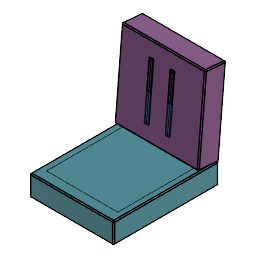
Smart_Chair (Autodesk Fusion 360 design; units mm, degrees)
part number: 2026-02-20-20-56-46-946
part number: 2026-02-20-20-58-49-113
part number: 2026-02-24-11-41-41-423
part number: 2026-02-24-11-48-27-673
part number: 2026-02-24-12-03-58-197
part number: 2026-02-24-12-17-04-515
Autodesk Fusion 360 part; units mm, degrees
sketch "Sketch1" plane through (0, 0, 0) normal (0, 0, 1) x (1, 0, 0) in component "Smart_Sprayer_Corner_Safety_Mount"
  line L0 (-12.6, 12.6) -> (12.6, 12.6) construction
  line L1 (12.6, 12.6) -> (12.6, -12.6) construction
  line L2 (12.6, -12.6) -> (-12.6, -12.6) construction
  line L3 (-12.6, -12.6) -> (-12.6, 12.6) construction
  line L4 (-12.6, 12.6) -> (12.6, -12.6) construction
  line L5 (12.6, 12.6) -> (-12.6, -12.6) construction
  line L6 (-12.6, 12.6) -> (-14.6, 12.6)
  line L7 (-14.6, 12.6) -> (-14.6, -12.6)
  line L8 (-14.6, -12.6) -> (-12.6, -12.6)
  line L9 (-12.6, -12.6) -> (-12.6, 12.6)
  line L10 (-14.6, -12.6) -> (12.6, -12.6)
  line L11 (12.6, -12.6) -> (12.6, -14.6)
  line L12 (12.6, -14.6) -> (-14.6, -14.6)
  line L13 (-14.6, -14.6) -> (-14.6, -12.6)
  dimension "d1" = 25.2
  dimension "d2" = 25.2
  dimension "d3" = 2
  dimension "d4" = 2
  constraint horizontal L0
  constraint perpendicular L0 L1
  constraint parallel L0 L2
  constraint parallel L1 L3
  constraint coincident L4 origin
  constraint coincident L5 origin
  constraint horizontal L6
  constraint vertical L7
  constraint horizontal L8
  constraint vertical L9
  constraint horizontal L10
  constraint vertical L11
  constraint horizontal L12
  constraint vertical L13
  measures "d1" distance of L1.end L2.end
  measures "d2" distance of L0.end L1.end
  measures "d3" distance of L0.start L6.end
  measures "d4" distance of L7.end L12.end
extrude "Extrude1" add sketch "Sketch1" along normal blind 27.2 makes body 1 in component "Smart_Sprayer_Corner_Safety_Mount"
sketch "Sketch2" plane through (0, -12.6, 0) normal (0, 1, 0) x (-1, 0, 0) in component "Smart_Sprayer_Corner_Safety_Mount"
  line L0 (-12.6, 0) -> (12.6, 0)
  line L1 (12.6, 0) -> (12.6, 27.2)
  line L2 (12.6, 27.2) -> (-12.6, 27.2)
  line L3 (-12.6, 27.2) -> (-12.6, 0)
  line L4 (-12.6, 27.2) -> (12.6, 27.2)
  line L5 (12.6, 27.2) -> (12.6, 25.2)
  line L6 (12.6, 25.2) -> (-12.6, 25.2)
  line L7 (-12.6, 25.2) -> (-12.6, 27.2)
  dimension "d7" = 2
  constraint horizontal L4
  constraint vertical L5
  constraint horizontal L6
  constraint vertical L7
  constraint coincident L2.end L3.start
  measures "d7" distance of L2.end L6.end
extrude "Extrude2" add sketch "Sketch2" along normal blind 25.2 contours L1 L2 L3 L4 L5 L6 L7 bodies 1 in component "Smart_Sprayer_Corner_Safety_Mount"
fillet "Fillet1" radius 1.25 9 edges at (-14.6, -1, 27.2) (-1, -14.6, 27.2) (-14.6, -14.6, 13.6) (12.6, -14.6, 13.6) (-1, 12.6, 27.2) (-14.6, -1, 0) (-14.6, 12.6, 13.6) (12.6, -1, 27.2) (-1, -14.6, 0) on bodies 1 in component "Smart_Sprayer_Corner_Safety_Mount"
sketch "Sketch1 (2)" plane through (0, 0, 0) normal (0, 1, 0) x (1, 0, 0) in component "Smart_Chair_Cushion_Back"
  line L0 (200, 200) -> (-200, 200)
  line L1 (-200, 200) -> (-200, -200)
  line L2 (-200, -200) -> (200, -200)
  line L3 (200, -200) -> (200, 200)
  line L4 (200, 200) -> (-200, -200) construction
  line L5 (-200, 200) -> (200, -200) construction
  dimension "d12" = 400
  dimension "d13" = 400
  constraint horizontal L0
  constraint perpendicular L0 L1
  constraint parallel L0 L2
  constraint parallel L1 L3
  constraint coincident L4 origin
  constraint coincident L5 origin
  measures "d12" distance of L1.end L2.end
  measures "d13" distance of L0.end L1.end
extrude "Extrude1'" add sketch "Sketch1 (2)" against normal blind 100 separate body makes body 2 in component "Smart_Chair_Cushion_Back"
fillet "Fillet1'" radius 5 6 faces at (-66.6667, -100, -66.6667) (-66.6667, -33.3333, 200) (200, -33.3333, 66.6667) (-66.6667, 0, -66.6667) (-200, -33.3333, -66.6667) (66.6667, -33.3333, -200) on bodies 2 in component "Smart_Chair_Cushion_Back"
sketch "Sketch1 (3)" plane through (0, -100, 0) normal (0, -1, 0) x (1, 0, 0) in component "Smart_Chair_Cushion_Back_Sensor_Mount"
  line L0 (195, 195) -> (-195, 195)
  line L1 (-195, 195) -> (-195, -195)
  line L2 (-195, -195) -> (195, -195)
  line L3 (195, -195) -> (195, 195)
  line L4 (-50, 195) -> (50, 195) construction
  line L5 (50, 195) -> (50, -195) construction
  line L6 (50, -195) -> (-50, -195) construction
  line L7 (-50, -195) -> (-50, 195) construction
  line L8 (-50, 195) -> (50, -195) construction
  line L9 (50, 195) -> (-50, -195) construction
  line L10 (0, 0) -> (0, 130) construction
  line L11 (0, 130) -> (-50, 130) construction
  line L12 (-50, 0) -> (-40, 0)
  line L13 (-40, 0) -> (-40, 130)
  line L14 (-40, 130) -> (-50, 130)
  line L15 (-50, 130) -> (-50, 0)
  line L16 (-50, 0) -> (-60, 0)
  line L17 (-60, 0) -> (-60, 130)
  line L18 (-60, 130) -> (-50, 130)
  line L19 (-50, 130) -> (-50, 0)
  dimension "d18" = 100
  dimension "d19" = 130
  dimension "d20" = 10
  dimension "d21" = 130
  dimension "d22" = 10
  dimension "d23" = 130
  constraint horizontal L4
  constraint perpendicular L4 L5
  constraint parallel L4 L6
  constraint parallel L5 L7
  constraint coincident L8 L10.start
  constraint coincident L9 L10.start
  constraint coincident L10.start origin
  constraint parallel L5 L10
  constraint coincident L7 L11.end
  constraint perpendicular L7 L11
  constraint horizontal L12
  constraint vertical L13
  constraint horizontal L14
  constraint vertical L15
  constraint midpoint L7 L12.start
  constraint horizontal L16
  constraint vertical L17
  constraint horizontal L18
  constraint vertical L19
  measures "d18" distance of L5.end L6.end
  measures "d19" distance of L10.start L10.end
  measures "d20" distance of L12.start L12.end
  measures "d21" distance of L12.start L11.end
  measures "d22" distance of L12.start L16.end
  measures "d23" distance of L12.start L11.end
extrude "Extrude1''" add sketch "Sketch1 (3)" along normal blind 3 separate body contours L12 L13 L14 L15 L19 | L15 L16 L17 L18 L19 makes body 3 in component "Smart_Chair_Cushion_Back_Sensor_Mount"
shell "Shell1" thickness 0.6 removed faces 2 at (-43.3333, -101, 130) at (-56.6667, -101, 130) on bodies 3 in component "Smart_Chair_Cushion_Back_Sensor_Mount"
sketch "Sketch2 (2)" plane through (0, -100, 0) normal (0, 1, 0) x (-1, 0, 0) in component "Smart_Chair_Cushion_Back_Sensor_Mount"
  line L0 (40, 0) -> (60, 0)
  line L1 (60, 0) -> (60, 130)
  line L2 (60, 130) -> (40, 130)
  line L3 (40, 130) -> (40, 0)
  line L4 (40, 130) -> (41, 130)
  line L5 (60, 130) -> (59, 130)
  line L6 (41, 130) -> (49, 130)
  line L7 (49, 130) -> (49, 0)
  line L8 (49, 0) -> (41, 0)
  line L9 (41, 0) -> (41, 130)
  line L10 (59, 130) -> (51, 130)
  line L11 (51, 130) -> (51, 0)
  line L12 (51, 0) -> (59, 0)
  line L13 (59, 0) -> (59, 130)
  dimension "d27" = 1
  dimension "d28" = 1
  dimension "d29" = 8
  dimension "d30" = 8
  constraint coincident L2.end L3.start
  constraint perpendicular L3 L4
  constraint coincident L1.end L2.start
  constraint perpendicular L1 L5
  constraint horizontal L6
  constraint vertical L7
  constraint horizontal L8
  constraint vertical L9
  constraint horizontal L10
  constraint vertical L11
  constraint horizontal L12
  constraint vertical L13
  measures "d27" distance of L2.end L4.end
  measures "d28" distance of L1.end L5.end
  measures "d29" distance of L4.end L6.end
  measures "d30" distance of L5.end L10.end
extrude "Extrude2'" add sketch "Sketch2 (2)" along normal blind 0.3 separate body contours L0 L2 L6 L7 L8 L9 | L0 L2 L10 L11 L12 L13 makes body 4 at (-43.6667, -100, 43.3333) makes body 5 at (-53.6667, -100, 43.3333) in component "Smart_Chair_Cushion_Back_Sensor_Mount"
chamfer "Chamfer1" distance 0.9 distance2 0.9 8 edges at (-40, -103, 65) (-40, -100, 65) (-40.6, -100.6, 65.3) (-40.6, -102.4, 65.3) (-59.4, -100.6, 65.3) (-59.4, -102.4, 65.3) (-60, -100, 65) (-60, -103, 65) measured on face at (-53.3333, -103, 86.6667) measured on face at (-40, -101, 43.3333) measured on face at (-53.1333, -100.6, 43.7333) measured on face at (-40.6, -101.8, 43.7333) measured on face at (-59.4, -101.8, 43.7333) measured on face at (-59.4, -101.8, 43.7333) measured on face at (-53.3333, -100, 86.6667) measured on face at (-53.3333, -103, 86.6667) on bodies 3 in component "Smart_Chair_Cushion_Back_Sensor_Mount"
sketch "Sketch3" plane through (0, -100, 0) normal (0, 1, 0) x (-1, 0, 0) in component "Smart_Chair_Cushion_Back_Sensor_Mount"
  line L0 (59.1, 0) -> (59.1, 130)
  line L1 (59.1, 130) -> (40.9, 130)
  line L2 (40.9, 130) -> (40.9, 0)
  line L3 (40.9, 0) -> (59.1, 0)
  line L4 (55, 125) -> (45, 125)
  line L5 (45, 125) -> (45, 135)
  line L6 (45, 135) -> (55, 135)
  line L7 (55, 135) -> (55, 125)
  line L8 (55, 125) -> (45, 135) construction
  line L9 (45, 125) -> (55, 135) construction
  point P0 (50, 130)
  dimension "d35" = 10
  dimension "d36" = 10
  constraint horizontal L4
  constraint perpendicular L4 L5
  constraint parallel L4 L6
  constraint parallel L5 L7
  constraint coincident L8 P0
  constraint coincident L9 P0
  constraint midpoint L1 P0
  measures "d35" distance of L5.end L6.end
  measures "d36" distance of L4.end L5.end
extrude "Extrude3" cut sketch "Sketch3" along normal mid plane 4 contours L1 L4 L5 L7 bodies 3 in component "Smart_Chair_Cushion_Back_Sensor_Mount"
pattern_linear "00000000-0000-0000-0000-000000000000" [suppressed]
sketch "Sketch1 (4)" plane through (0, -100, 0) normal (0, -1, 0) x (1, 0, 0) in component "Smart_Chair_Cushion_Back_Sensor_Mount (1)"
  line L0 (195, 195) -> (-195, 195)
  line L1 (-195, 195) -> (-195, -195)
  line L2 (-195, -195) -> (195, -195)
  line L3 (195, -195) -> (195, 195)
  line L4 (-50, 195) -> (50, 195) construction
  line L5 (50, 195) -> (50, -195) construction
  line L6 (50, -195) -> (-50, -195) construction
  line L7 (-50, -195) -> (-50, 195) construction
  line L8 (-50, 195) -> (50, -195) construction
  line L9 (50, 195) -> (-50, -195) construction
  line L10 (0, 0) -> (0, 130) construction
  line L11 (0, 130) -> (-50, 130) construction
  line L12 (-50, 0) -> (-40, 0)
  line L13 (-40, 0) -> (-40, 130)
  line L14 (-40, 130) -> (-50, 130)
  line L15 (-50, 130) -> (-50, 0)
  line L16 (-50, 0) -> (-60, 0)
  line L17 (-60, 0) -> (-60, 130)
  line L18 (-60, 130) -> (-50, 130)
  line L19 (-50, 130) -> (-50, 0)
  dimension "d18_1" = 100
  dimension "d19_1" = 130
  dimension "d20_1" = 10
  dimension "d21_1" = 130
  dimension "d22_1" = 10
  dimension "d23_1" = 130
  constraint horizontal L4
  constraint perpendicular L4 L5
  constraint parallel L4 L6
  constraint parallel L5 L7
  constraint coincident L8 L10.start
  constraint coincident L9 L10.start
  constraint coincident L10.start origin
  constraint parallel L5 L10
  constraint coincident L7 L11.end
  constraint perpendicular L7 L11
  constraint horizontal L12
  constraint vertical L13
  constraint horizontal L14
  constraint vertical L15
  constraint midpoint L7 L12.start
  constraint horizontal L16
  constraint vertical L17
  constraint horizontal L18
  constraint vertical L19
  measures "d18_1" distance of L5.end L6.end
  measures "d19_1" distance of L10.start L10.end
  measures "d20_1" distance of L12.start L12.end
  measures "d21_1" distance of L12.start L11.end
  measures "d22_1" distance of L12.start L16.end
  measures "d23_1" distance of L12.start L11.end
extrude "Extrude1'''" add sketch "Sketch1 (4)" along normal blind 3 separate body contours L12 L13 L14 L15 L19 | L15 L16 L17 L18 L19 makes body 6 in component "Smart_Chair_Cushion_Back_Sensor_Mount (1)"
shell "Shell1'" thickness 0.6 removed faces 2 at (-43.3333, -101, 130) at (-56.6667, -101, 130) on bodies 6 in component "Smart_Chair_Cushion_Back_Sensor_Mount (1)"
sketch "Sketch2 (3)" plane through (0, -100, 0) normal (0, 1, 0) x (-1, 0, 0) in component "Smart_Chair_Cushion_Back_Sensor_Mount (1)"
  line L0 (40, 0) -> (60, 0)
  line L1 (60, 0) -> (60, 130)
  line L2 (60, 130) -> (40, 130)
  line L3 (40, 130) -> (40, 0)
  line L4 (40, 130) -> (41, 130)
  line L5 (60, 130) -> (59, 130)
  line L6 (41, 130) -> (49, 130)
  line L7 (49, 130) -> (49, 0)
  line L8 (49, 0) -> (41, 0)
  line L9 (41, 0) -> (41, 130)
  line L10 (59, 130) -> (51, 130)
  line L11 (51, 130) -> (51, 0)
  line L12 (51, 0) -> (59, 0)
  line L13 (59, 0) -> (59, 130)
  dimension "d27_1" = 1
  dimension "d28_1" = 1
  dimension "d29_1" = 8
  dimension "d30_1" = 8
  constraint coincident L2.end L3.start
  constraint perpendicular L3 L4
  constraint coincident L1.end L2.start
  constraint perpendicular L1 L5
  constraint horizontal L6
  constraint vertical L7
  constraint horizontal L8
  constraint vertical L9
  constraint horizontal L10
  constraint vertical L11
  constraint horizontal L12
  constraint vertical L13
  measures "d27_1" distance of L2.end L4.end
  measures "d28_1" distance of L1.end L5.end
  measures "d29_1" distance of L4.end L6.end
  measures "d30_1" distance of L5.end L10.end
extrude "Extrude2''" add sketch "Sketch2 (3)" along normal blind 0.3 separate body contours L0 L2 L6 L7 L8 L9 | L0 L2 L10 L11 L12 L13 makes body 7 at (-43.6667, -100, 43.3333) makes body 8 at (-53.6667, -100, 43.3333) in component "Smart_Chair_Cushion_Back_Sensor_Mount (1)"
chamfer "Chamfer1'" distance 0.9 distance2 0.9 8 edges at (-40, -103, 65) (-40, -100, 65) (-40.6, -100.6, 65.3) (-40.6, -102.4, 65.3) (-59.4, -100.6, 65.3) (-59.4, -102.4, 65.3) (-60, -100, 65) (-60, -103, 65) measured on face at (-53.3333, -103, 86.6667) measured on face at (-40, -101, 43.3333) measured on face at (-53.1333, -100.6, 43.7333) measured on face at (-40.6, -101.8, 43.7333) measured on face at (-59.4, -101.8, 43.7333) measured on face at (-59.4, -101.8, 43.7333) measured on face at (-53.3333, -100, 86.6667) measured on face at (-53.3333, -103, 86.6667) on bodies 6 in component "Smart_Chair_Cushion_Back_Sensor_Mount (1)"
sketch "Sketch3 (2)" plane through (0, -100, 0) normal (0, 1, 0) x (-1, 0, 0) in component "Smart_Chair_Cushion_Back_Sensor_Mount (1)"
  line L0 (59.1, 0) -> (59.1, 130)
  line L1 (59.1, 130) -> (40.9, 130)
  line L2 (40.9, 130) -> (40.9, 0)
  line L3 (40.9, 0) -> (59.1, 0)
  line L4 (55, 125) -> (45, 125)
  line L5 (45, 125) -> (45, 135)
  line L6 (45, 135) -> (55, 135)
  line L7 (55, 135) -> (55, 125)
  line L8 (55, 125) -> (45, 135) construction
  line L9 (45, 125) -> (55, 135) construction
  point P0 (50, 130)
  dimension "d35_1" = 10
  dimension "d36_1" = 10
  constraint horizontal L4
  constraint perpendicular L4 L5
  constraint parallel L4 L6
  constraint parallel L5 L7
  constraint coincident L8 P0
  constraint coincident L9 P0
  constraint midpoint L1 P0
  measures "d35_1" distance of L5.end L6.end
  measures "d36_1" distance of L4.end L5.end
extrude "Extrude3'" cut sketch "Sketch3 (2)" along normal mid plane 4 contours L1 L4 L5 L7 bodies 6 in component "Smart_Chair_Cushion_Back_Sensor_Mount (1)"
sketch "Sketch4" plane through (0, -103, 0) normal (0, -1, 0) x (1, 0, 0) in component "Smart_Chair_Cushion_Back_Sensor_Mount (1)"
  line L0 (-59.1, 130) -> (-59.1, 0)
  line L1 (-59.1, 0) -> (-40.9, 0)
  line L2 (-40.9, 0) -> (-40.9, 130)
  line L3 (-40.9, 130) -> (-59.1, 130)
pattern_linear "00000000-0000-0000-0000-000000000000'" [suppressed]
sketch "Sketch2 (4)" plane through (0, -100, 0) normal (0, -1, 0) x (1, 0, 0) in component "Smart_Chair_Cushion_Back"
  line L0 (195, 195) -> (-195, 195)
  line L1 (-195, 195) -> (-195, -195)
  line L2 (-195, -195) -> (195, -195)
  line L3 (195, -195) -> (195, 195)
  line L4 (-50, 195) -> (50, 195) construction
  line L5 (50, 195) -> (50, -195) construction
  line L6 (50, -195) -> (-50, -195) construction
  line L7 (-50, -195) -> (-50, 195) construction
  line L8 (-50, 195) -> (50, -195) construction
  line L9 (50, 195) -> (-50, -195) construction
  line L10 (-47.1154, 122.5) -> (47.1154, 122.5) construction
  line L11 (47.1154, 122.5) -> (47.1154, -122.5) construction
  line L12 (47.1154, -122.5) -> (-47.1154, -122.5) construction
  line L13 (-47.1154, -122.5) -> (-47.1154, 122.5) construction
  line L14 (-47.1154, 122.5) -> (47.1154, -122.5) construction
  line L15 (47.1154, 122.5) -> (-47.1154, -122.5) construction
  circle A0 centre (-50, 122.5) radius 2
  circle A1 centre (50, 122.5) radius 2
  circle A2 centre (-50, -122.5) radius 2
  circle A3 centre (50, -122.5) radius 2
  dimension "d47" = 100
  dimension "d48" = 245
  dimension "d49" = 4
  dimension "d50" = 4
  dimension "d51" = 4
  dimension "d52" = 4
  constraint horizontal L4
  constraint perpendicular L4 L5
  constraint parallel L4 L6
  constraint parallel L5 L7
  constraint coincident L8 origin
  constraint coincident L9 origin
  constraint horizontal L10
  constraint perpendicular L10 L11
  constraint parallel L10 L12
  constraint parallel L11 L13
  constraint coincident L14 origin
  constraint coincident L15 origin
  constraint coincident L7 A0.centre
  constraint coincident L5 A1.centre
  constraint coincident L7 A2.centre
  constraint coincident L5 A3.centre
  measures "d47" distance of L5.end L6.end
  measures "d48" distance of L10.end L11.end
  measures "d49" diameter of A0
  measures "d50" diameter of A1
  measures "d51" diameter of A2
  measures "d52" diameter of A3
extrude "Extrude2'''" cut sketch "Sketch2 (4)" against normal blind 10 contours A0 | A1 | A2 | A3 bodies 2 in component "Smart_Chair_Cushion_Back"
sketch "Sketch3 (3)" plane through (0, 0, 0) normal (1, 0, 0) x (0, 1, 0) in component "Smart_Chair_Cushion_Back"
sketch "Sketch4 (2)" plane through (-200, 0, 0) normal (-1, 0, 0) x (0, -1, 0) in component "Smart_Chair_Cushion_Back"
  line L0 (5, -195) -> (95, -195)
  line L1 (95, -195) -> (95, 195)
  line L2 (95, 195) -> (5, 195)
  line L3 (5, 195) -> (5, -195)
  line L4 (50, 195) -> (50, 95) construction
  line L5 (50, -195) -> (50, -95) construction
  circle A0 centre (50, -95) radius 2 construction
  circle A1 centre (50, 95) radius 2
  circle A2 centre (50, -95) radius 2
  dimension "d55" = 100
  dimension "d56" = 100
  dimension "d57" = 4
  dimension "d58" = 4
  dimension "d59" = 4
  constraint vertical L4
  constraint midpoint L2 L4.start
  constraint midpoint L0 L5.start
  constraint perpendicular L0 L5
  constraint coincident L5.end A0.centre
  constraint coincident L4.end A1.centre
  measures "d55" distance of L4.start L4.end
  measures "d56" distance of L5.start L5.end
  measures "d57" diameter of A0
  measures "d58" diameter of A1
  measures "d59" diameter of A2
extrude "Extrude3''" cut sketch "Sketch4 (2)" against normal blind 10 contours A1 | A2 bodies 2 in component "Smart_Chair_Cushion_Back"
sketch "Sketch5" plane through (-200, 0, 0) normal (-1, 0, 0) x (0, -1, 0) in component "Smart_Chair_Cushion_Back"
  circle A0 centre (50, 95) radius 2
  circle A1 centre (50, -95) radius 2
  line L0 (5, -195) -> (95, -195)
  line L1 (95, -195) -> (95, 195)
  line L2 (95, 195) -> (5, 195)
  line L3 (5, 195) -> (5, -195)
  line L4 (50, 95) -> (50, -95) construction
  line L5 (0, 50) -> (100, 50) construction
  line L6 (100, 50) -> (100, -50) construction
  line L7 (100, -50) -> (0, -50) construction
  line L8 (0, -50) -> (0, 50) construction
  line L9 (0, 50) -> (100, -50) construction
  line L10 (100, 50) -> (0, -50) construction
  line L11 (20, 50) -> (80, 50) construction
  line L12 (80, 50) -> (80, -50) construction
  line L13 (80, -50) -> (20, -50) construction
  line L14 (20, -50) -> (20, 50) construction
  line L15 (20, 50) -> (80, -50) construction
  line L16 (80, 50) -> (20, -50) construction
  line L17 (20, 50) -> (30, 50)
  line L18 (30, 50) -> (30, -50)
  line L19 (30, -50) -> (20, -50)
  line L20 (20, -50) -> (20, 50)
  line L21 (20, 50) -> (10, 50)
  line L22 (10, 50) -> (10, -50)
  line L23 (10, -50) -> (20, -50)
  line L24 (20, -50) -> (20, 50)
  line L25 (80, 50) -> (70, 50)
  line L26 (70, 50) -> (70, -50)
  line L27 (70, -50) -> (80, -50)
  line L28 (80, -50) -> (80, 50)
  line L29 (80, 50) -> (90, 50)
  line L30 (90, 50) -> (90, -50)
  line L31 (90, -50) -> (80, -50)
  line L32 (80, -50) -> (80, 50)
  point P0 (50, 0)
  point P1 (50, 0)
  dimension "d62" = 100
  dimension "d63" = 100
  dimension "d64" = 60
  dimension "d65" = 10
  constraint coincident A0.centre L4.start
  constraint coincident A1.centre L4.end
  constraint horizontal L5
  constraint perpendicular L5 L6
  constraint parallel L5 L7
  constraint parallel L6 L8
  constraint coincident L9 P1
  constraint coincident L10 P1
  constraint midpoint L4 P1
  constraint horizontal L11
  constraint perpendicular L11 L12
  constraint parallel L11 L13
  constraint parallel L12 L14
  constraint coincident L15 P1
  constraint coincident L16 P1
  constraint coincident P1 P0
  constraint horizontal L17
  constraint vertical L18
  constraint horizontal L19
  constraint vertical L20
  constraint horizontal L21
  constraint vertical L22
  constraint horizontal L23
  constraint vertical L24
  constraint coincident L7 L22.end
  constraint horizontal L25
  constraint vertical L26
  constraint horizontal L27
  constraint vertical L28
  constraint coincident L7 L26.end
  constraint horizontal L29
  constraint vertical L30
  constraint horizontal L31
  constraint vertical L32
  constraint coincident L7 L30.end
  measures "d62" distance of L6.end L7.end
  measures "d63" distance of L5.end L6.end
  measures "d64" distance of L12.end L13.end
  measures "d65" distance of L11.start L17.end
extrude "Extrude4" add sketch "Sketch5" along normal blind 0.3 separate body contours L17 L18 L19 L20 L24 | L20 L21 L22 L23 L24 | L25 L26 L27 L28 L32 | L28 L29 L30 L31 L32 makes body 9 at (-200, -16.6667, 16.6667) makes body 10 at (-200, -83.3333, -16.6667) in component "Smart_Chair_Cushion_Back"
sketch "Sketch1 (5)" plane through (0, 0, 0) normal (0, 0, 1) x (1, 0, 0) in component "Smart_Chair_Cushion_Sit"
  line L0 (0, -120) -> (0, -520) construction
  line L1 (-200, -520) -> (200, -520)
  line L2 (200, -520) -> (200, -120)
  line L3 (200, -120) -> (-200, -120)
  line L4 (-200, -120) -> (-200, -520)
  line L5 (-200, -520) -> (200, -120) construction
  line L6 (200, -520) -> (-200, -120) construction
  point P0 (0, -320)
  dimension "d68" = 400
  dimension "d69" = 400
  dimension "d70" = 400
  constraint vertical L0
  constraint horizontal L1
  constraint perpendicular L1 L2
  constraint parallel L1 L3
  constraint parallel L2 L4
  constraint coincident L5 P0
  constraint coincident L6 P0
  constraint midpoint L0 P0
  measures "d68" distance of L0.start L0.end
  measures "d69" distance of L2.end L3.end
  measures "d70" distance of L1.end L2.end
extrude "Extrude1''''" add sketch "Sketch1 (5)" against normal blind 300 separate body makes body 11 in component "Smart_Chair_Cushion_Sit"
extrude "Extrude2''''" cut 1 faces at (-66.6667, -253.3333, 0) along direction (0, 0, -1) blind 200 on bodies 11 bodies 11 in component "Smart_Chair_Cushion_Sit"
extrude "Extrude3'''" add 1 faces at (66.6667, -120, -233.3333) along direction (0, 1, 0) blind 100 on bodies 11 bodies 11 in component "Smart_Chair_Cushion_Sit"
fillet "Fillet1''" radius 5 1 edges at (-200, -270, -300) 6 faces at (200, -186.6667, -266.6667) (66.6667, -20, -233.3333) (-66.6667, -520, -233.3333) (-66.6667, -186.6667, -200) (-200, -353.3333, -233.3333) (-66.6667, -186.6667, -300) on bodies 11 in component "Smart_Chair_Cushion_Sit"
sketch "Sketch2 (5)" plane through (0, 0, -300) normal (0, 0, -1) x (1, 0, 0) in component "Smart_Chair_Cushion_Sit"
  line L0 (-195, 515) -> (-195, 25)
  line L1 (-195, 25) -> (195, 25)
  line L2 (195, 25) -> (195, 515)
  line L3 (195, 515) -> (-195, 515)
  line L4 (-195, 515) -> (195, 25) construction
  line L5 (-170, 470) -> (170, 470)
  line L6 (170, 470) -> (170, 70)
  line L7 (170, 70) -> (-170, 70)
  line L8 (-170, 70) -> (-170, 470)
  line L9 (-170, 470) -> (170, 70) construction
  line L10 (170, 470) -> (-170, 70) construction
  point P0 (0, 270)
  dimension "d79" = 340
  dimension "d80" = 400
  constraint coincident L0.start L3.end
  constraint coincident L1.end L2.start
  constraint horizontal L5
  constraint perpendicular L5 L6
  constraint parallel L5 L7
  constraint parallel L6 L8
  constraint coincident L9 P0
  constraint coincident L10 P0
  constraint midpoint L4 P0
  measures "d79" distance of L6.end L7.end
  measures "d80" distance of L5.end L6.end
extrude "Extrude4'" cut sketch "Sketch2 (5)" against normal blind 97 contours L5 L6 L7 L8 bodies 11 in component "Smart_Chair_Cushion_Sit"
component "Smart_Sprayer_Corner_Safety_Mount" placed x (1, 0, 0) y (0, 1, 0) z (0, 0, 1) at (0, 0, 0)
component "Smart_Chair_Cushion_Back" placed x (1, 0, 0) y (0, 0.996195, -0.087156) z (0, 0.087156, 0.996195) at (0, -0.1904, -4.3619)
component "Smart_Chair_Cushion_Back_Sensor_Mount" placed x (1, 0, 0) y (0, 0.996195, -0.087156) z (0, 0.087156, 0.996195) at (0, -0.1904, -4.3619)
component "Smart_Chair_Cushion_Back_Sensor_Mount" placed x (1, 0, 0) y (0, 0.996195, -0.087156) z (0, 0.087156, 0.996195) at (100, -0.1904, -4.3619)
component "Smart_Chair_Cushion_Back_Sensor_Mount (1)" placed x (-1, 0, 0) y (0, 0.996195, -0.087156) z (0, -0.087156, -0.996195) at (0, -0.3287, -5.9423)
component "Smart_Chair_Cushion_Back_Sensor_Mount (1)" placed x (-1, 0, 0) y (0, 0.996195, -0.087156) z (0, -0.087156, -0.996195) at (-100, -0.3287, -5.9423)
component "Smart_Chair_Cushion_Sit" placed x (1, 0, 0) y (0, 1, 0) z (0, 0, 1) at (0, 0, 0)
